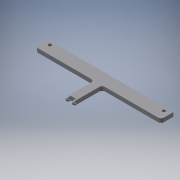
# Autodesk Inventor part: WebcamBase
Saved by Autodesk Inventor 2017 (Build 210142000, 142)
## iProperties
Created: 2015-05-12
Part Number: WebcamBase
Material: Generic
Document SubType Name: Modeling
Designer: Kurtis
Density: 1 g/cm^3
Appearance: Default
Author: Kurtis
Autodesk Inventor part; units mm, degrees
ref_plane "YZ Plane" through (0, 0, 0) normal (1, 0, 0) x (0, 1, 0)
ref_plane "XZ Plane" through (0, 0, 0) normal (0, 1, 0) x (-1, 0, 0)
ref_plane "XY Plane" through (0, 0, 0) normal (0, 0, 1) x (1, 0, 0)
sketch "Sketch1" plane through (0, 0, 0) normal (0, 0, 1) x (1, 0, 0)
  line L0 (254, 0) -> (254, 25)
  line L1 (254, 25) -> (0, 25)
  line L2 (0, 25) -> (0, 0)
  line L3 (0, 25) -> (0, 21) construction
  line L4 (0, 21) -> (8.5, 21) construction
  line L5 (8.5, 21) -> (11.75, 21) construction
  line L6 (11.75, 21) -> (11.75, 17.75) construction
  circle A0 centre (11.75, 17.75) radius 3.25
  line L7 (254, 25) -> (254, 21) construction
  line L8 (254, 21) -> (245.5, 21) construction
  line L9 (245.5, 21) -> (245.5, 17.75) construction
  line L10 (245.5, 17.75) -> (242.25, 17.75) construction
  circle A1 centre (242.25, 17.75) radius 3.25
  line L11 (0, 0) -> (254, 0)
  line L12 (127, 0) -> (127, -50) construction
  line L13 (122, -50) -> (132, -50)
  line L14 (132, -50) -> (132, -58)
  line L15 (122, -50) -> (122, -58)
  line L16 (132, -58) -> (135, -58)
  line L17 (122, -58) -> (119, -58)
  line L18 (119, -58) -> (119, 0)
  line L19 (135, -58) -> (135, 0)
  dimension "d1" = 25
  dimension "d2" = 4
  dimension "d3" = 8.5
  dimension "d4" = 3.25
  dimension "d5" = 3.25
  dimension "d6" = 4
  dimension "d7" = 8.5
  dimension "d8" = 3.25
  dimension "d9" = 3.25
  dimension "d14" = 242.25
  dimension "d40" = 50
  dimension "d41" = 10
  dimension "d42" = 5
  dimension "d43" = 0
  dimension "d44" = 8
  dimension "d45" = 8
  dimension "d46" = 3
  dimension "d47" = 3
  constraints: 40 end point, 7 perpendicular, 5 horizontal, 5 point on line, 4 vertical, 2 coincident, 1 horizontal alignment, 1 midpoint, 1 vertical alignment, 4 other
  measures "d1" distance of L0.start L0.end
  measures "d2" distance of L1.end L3.end
  measures "d3" distance of L3.end L4.end
  measures "d4" distance of L4.end L5.end
  measures "d5" distance of L5.end L6.end
  measures "d6" distance of L0.end L7.end
  measures "d7" distance of L7.end L8.end
  measures "d8" distance of L8.end L9.end
  measures "d9" distance of L9.end L10.end
  measures "d14" distance between parallel lines of L6 L0
  measures "d40" distance of L12.start L12.end
  measures "d41" distance of L13.start L13.end
  measures "d42" distance of L12.end L13.end
  measures "d43" distance from line of L12.end L13
  measures "d44" distance of L13.end L14.end
  measures "d45" distance of L13.start L15.end
  measures "d46" distance of L14.end L16.end
  measures "d47" distance of L15.end L17.end
extrude "Extrusion1" add sketch "Sketch1" along normal blind 8
fillet "Fillet2" radius 4 4 edges at (120.5, -58, 8) (120.5, -58, 0) (133.5, -58, 0) (133.5, -58, 8)
fillet "Fillet4" radius 6 4 edges at (0, 0, 4) (254, 0, 4) (135, 0, 4) (119, 0, 4)
hole "Hole1" at (135, -54, 4) direction (-1, 0, 0) diameter 3 end through all
equation "\"d42\" = 0.5 * d41"
equation "\"d45\" = d44"
equation "\"d47\" = d46"
body "Solid1"
